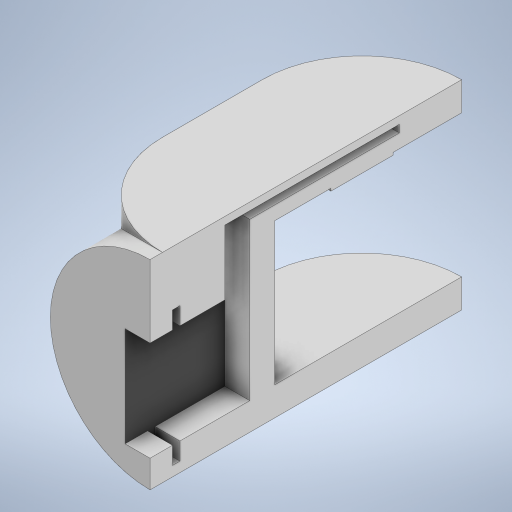
# Autodesk Inventor part: wirst 1 right
Saved by Autodesk Inventor 2023 (Build 270158000, 158)
## iProperties
Created: 2024-06-28
Part Number: wirst 1 right
Material: Generic
Document SubType Name: Modeling
Designer: Swoby
Density: 1 g/cm^3
Appearance: Default
Author: Swoby
Autodesk Inventor part; units mm, degrees
ref_plane "YZ Plane" through (0, 0, 0) normal (1, 0, 0) x (0, 1, 0)
ref_plane "XZ Plane" through (0, 0, 0) normal (0, 1, 0) x (-1, 0, 0)
ref_plane "XY Plane" through (0, 0, 0) normal (0, 0, 1) x (1, 0, 0)
sketch "Sketch1" plane through (0, 0, 0) normal (0, 0, 1) x (1, 0, 0)
  line L0 (-10, -36) -> (10, -36) construction
  line L1 (10, -36) -> (10, 18) construction
  line L2 (10, 18) -> (-10, 18) construction
  line L3 (-10, 18) -> (-10, -36) construction
  line L4 (-10, -36) -> (10, 18) construction
  line L5 (10, -36) -> (-10, 18) construction
  circle A0 centre (0, 0) radius 2.5 construction
  line L6 (-10, -29) -> (10, -29) construction
  line L7 (10, -29) -> (10, 11) construction
  line L8 (10, 11) -> (-10, 11) construction
  line L9 (-10, 11) -> (-10, -29) construction
  line L10 (-10, -29) -> (10, 11) construction
  line L11 (10, -29) -> (-10, 11) construction
  line L12 (0, 26.4398) -> (0, -41)
  arc A1 (0, 40) -> (0, -40) centre (0, 0) ccw
  line L13 (0, 40) -> (0, -40)
  point P0 (0, -9)
  point P1 (0, -9)
  dimension "d0" = 5
  dimension "d1" = 20
  dimension "d2" = 54
  dimension "d3" = 36
  dimension "d4" = 40
  dimension "d5" = 7
  dimension "d27" = 80
  constraints: 28 end point, 5 midpoint, 4 parallel, 4 point on line, 2 centre point, 2 coincident, 2 horizontal, 2 perpendicular, 2 point on circle, 1 collinear, 1 vertical
  measures "d0" diameter of A0
  measures "d1" distance of L1.end L2.end
  measures "d2" distance of L0.end L1.end
  measures "d3" distance from line of L0 point (0, 0)
  measures "d4" distance of L7.end L6.end
  measures "d5" distance between parallel lines of L8 L2
  measures "d27" diameter of A1
sketch "Sketch3" plane through (0, 0, 0) normal (1, 0, 0) x (0, 1, 0)
  line L0 (0, 0) -> (0, -69)
  line L1 (0, 0) -> (40, 0)
  line L2 (40, 0) -> (40, -45)
  line L3 (40, -45) -> (37.5, -50)
  line L4 (37.5, -50) -> (0, -50)
  dimension "d28" = 40
  dimension "d29" = 45
  dimension "d30" = 75
  dimension "d31" = 5
  constraints: 10 end point, 2 vertical, 1 horizontal, 1 perpendicular, 1 point on line
  measures "d28" distance of L0.start L1.end
  measures "d29" distance of L1.end L2.end
  measures "d30" diameter of L3.end L0
  measures "d31" vertical distance of L2.end L3.end
revolve "Revolution1" add sketch "Sketch3" angle 180 about axis through (0, 0, 0) along (0, 0, 1)
sketch "Sketch4" plane through (0, -37.5, -50) normal (0, 0, -1) x (-1, 0, 0)
  line L0 (0, 0) -> (0, 75) projected
  line L1 (0, 75) -> (0, 77.5) projected
  line L2 (0, -2.5) -> (0, 0) projected
  line L3 (0, 66) -> (40, 66)
  line L4 (40, 66) -> (40, 77.5)
  line L5 (40, 77.5) -> (0, 77.5)
  line L6 (0, 77.5) -> (0, 66)
  line L7 (0, -2.5) -> (40, -2.5)
  line L8 (40, -2.5) -> (40, 9)
  line L9 (40, 9) -> (0, 9)
  line L10 (0, 9) -> (0, -2.5)
  point P0 (0, 37.5)
  dimension "d33" = 11.5
  dimension "d34" = 40
  dimension "d35" = 11.5
  constraints: 16 end point, 3 perpendicular, 2 collinear, 2 horizontal, 2 parallel, 1 point on line
  measures "d33" distance of L3.end L4.end
  measures "d34" distance of L4.end L1.end
  measures "d35" distance of L7.end L8.end
extrude "Extrusion2" add sketch "Sketch4" along normal blind 75 and the other way blind 5
sketch "Sketch5" plane through (-40, 40, -125) normal (0, 1, 0) x (1, 0, 0)
  line L0 (0, -80) -> (0, 0) projected
  line L1 (11.9331, -80) -> (40, -80) projected
  line L2 (0, -80) -> (40, -80)
  line L3 (0, -125) -> (40, -125) projected
  line L4 (40, -80) -> (40, -120)
  arc A0 (0, -80) -> (40, -120) centre (40, -80) ccw
  line L5 (40, -80) -> (40, -125) projected
  dimension "d42" = 40
  constraints: 4 end point, 2 point on circle, 1 centre point, 1 horizontal, 1 point on line, 1 tangent
  measures "d42" distance of L1.end L4.end
extrude "Extrusion3" add sketch "Sketch5" against normal up to surface (11.5 mm away)
sketch "Sketch6" plane through (-40, -40, -125) normal (0, -1, 0) x (1, 0, 0)
  arc A0 (40, 120) -> (0, 80) centre (40, 80) ccw projected
  line L0 (40, 0) -> (40, 120) projected
  line L1 (0, 0) -> (40, 0) projected
  line L2 (0, 80) -> (0, 0) projected
  arc A1 (40, 120) -> (0, 80) centre (40, 80) ccw projected
  point P0 (40, 125)
  point P1 (0, 80)
extrude "Extrusion4" add sketch "Sketch6" against normal up to surface (11.5 mm away)
sketch "Sketch7" plane through (-40, 40, -125) normal (0, 1, 0) x (1, 0, 0)
  line L0 (0, 0) -> (40, 0) projected
  line L1 (0, 0) -> (0, -80) projected
  arc A0 (40, 0) -> (0, -40) centre (40, -40) ccw
  line L2 (0, -40) -> (0, 0)
  line L3 (40, 0) -> (0, 0)
  line L4 (0, 0) -> (40, 0) projected
  point P0 (40, -125)
  constraints: 4 end point, 2 perpendicular, 2 point on circle, 2 tangent, 1 centre point, 1 midpoint
extrude "Extrusion5" cut sketch "Sketch7" along normal through all both and the other way through all
sketch "Sketch8" plane through (0, -40, 0) normal (1, 0, 0) x (0, 0, -1)
  line L0 (0, 58) -> (40, 58) construction
  line L1 (40, 58) -> (40, 51) construction
  line L2 (40, 4) -> (0, 4) construction
  line L3 (0, 4) -> (0, 58)
  line L4 (0, 51) -> (9, 51)
  line L5 (0, 11) -> (9, 11)
  line L6 (0, 80) -> (0, 0) projected
  line L7 (0, 42.5) -> (0, 37.5) construction
  line L8 (0, 37.5) -> (-5, 37.5)
  line L9 (-5, 37.5) -> (-5, 42.5)
  line L10 (-5, 42.5) -> (0, 42.5)
  line L11 (0, 42.5) -> (0, 37.5)
  line L12 (40, 51) -> (40, 11)
  line L13 (40, 11) -> (40, 4) construction
  line L14 (9, 51) -> (12, 51) construction
  line L15 (12, 51) -> (12, 58)
  line L16 (12, 58) -> (9, 58)
  line L17 (9, 58) -> (9, 51)
  line L18 (9, 11) -> (12, 11) construction
  line L19 (12, 11) -> (12, 4)
  line L20 (12, 4) -> (9, 4)
  line L21 (9, 4) -> (9, 11)
  line L22 (32, 51) -> (32, 56)
  line L23 (32, 56) -> (35, 56)
  line L24 (35, 56) -> (35, 51)
  line L25 (125, 80) -> (85, 80) projected
  line L26 (40, 51) -> (35, 51)
  line L27 (30, 51) -> (30, 77)
  line L28 (30, 77) -> (40, 77)
  line L29 (40, 77) -> (40, 51)
  line L30 (12, 51) -> (30, 51)
  line L31 (9, 51) -> (12, 51) construction
  line L32 (30, 51) -> (32, 51)
  line L33 (9, 11) -> (12, 11) construction
  line L34 (12, 11) -> (40, 11)
  line L35 (35, 51) -> (32, 51) construction
  line L36 (32, 51) -> (35, 51) construction
  line L37 (32, 51) -> (30, 51)
  line L38 (125, 80) -> (5, 80) projected
  line L39 (40, 77) -> (100, 77)
  line L40 (100, 77) -> (100, 74)
  line L41 (100, 74) -> (40, 74)
  line L42 (40, 74) -> (40, 77)
  line L43 (85, 80) -> (85, 68.5) projected
  line L44 (35, 51) -> (40, 51)
  point P0 (0, 40)
  point P1 (0, 40)
  point P2 (0, 4)
  point P3 (35, 77)
  dimension "d47" = 40
  dimension "d48" = 5
  dimension "d49" = 5
  dimension "d50" = 3
  dimension "d51" = 9
  dimension "d52" = 3
  dimension "d53" = 5
  dimension "d54" = 5
  dimension "d55" = 10
  dimension "d56" = 3
  dimension "d57" = 60
  dimension "d58" = 3
  constraints: 80 end point, 35 perpendicular, 34 parallel, 11 point on line, 8 horizontal, 1 midpoint, 1 vertical, 1 other
  measures "d47" distance of L0.start L0.end
  measures "d48" distance of L8.end L9.end
  measures "d49" distance of L9.end L10.end
  measures "d50" distance of L15.end L16.end
  measures "d51" distance between parallel lines of L3 L17
  measures "d52" distance of L22.end L23.end
  measures "d53" distance of L22.start L22.end
  measures "d54" distance between parallel lines of L12 L24
  measures "d55" distance of L27.end L28.end
  measures "d56" distance from line of point (35, 77) L38
  measures "d57" distance of L28.end L39.end
  measures "d58" distance of L39.end L40.end
extrude "Extrusion6" cut sketch "Sketch8" against normal blind 10 contours L3 L4 L17 L16 L15 L30 L32 L22 L23 L24 L26 L12 L34 L19 L20 L21 L5 | L26 L24 L23 L22 L32 L27 L28 L29 | L29 L39 L43 L41 | L43 L39 L40 L41
sketch "Sketch9" plane through (-24.3721, 28.5, -50) normal (0, -1, 0) x (1, 0, 0)
  arc A0 (-15.6279, -35) -> (24.3721, -75) centre (24.3721, -35) ccw projected
  arc A1 (24.3721, -22.5) -> (24.3721, -47.5) centre (24.3721, -35) ccw
  line L0 (24.3721, -50) -> (24.3721, 10) projected
  line L1 (24.3721, -22.5) -> (24.3721, -47.5)
  point P0 (24.3721, 50)
  dimension "d61" = 25
  constraints: 2 end point, 2 point on circle, 2 point on line, 1 centre point, 1 coincident
  measures "d61" diameter of A1
extrude "Extrusion7" add sketch "Sketch9" along normal blind 1
equation "\"d35\" = d33"
body "Solid2"
